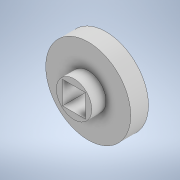
# Autodesk Inventor part: secondwheel
Saved by Autodesk Inventor 2020 (Build 240168000, 168)
## iProperties
Created: 2021-01-09
Part Number: secondwheel
Material: Generic
Document SubType Name: Modeling
Designer: papa
Density: 1 g/cm^3
Appearance: Default
Author: papa
Autodesk Inventor part; units mm, degrees
ref_plane "YZ Plane" through (0, 0, 0) normal (1, 0, 0) x (0, 1, 0)
ref_plane "XZ Plane" through (0, 0, 0) normal (0, 1, 0) x (-1, 0, 0)
ref_plane "XY Plane" through (0, 0, 0) normal (0, 0, 1) x (1, 0, 0)
sketch "Sketch1" plane through (0, 0, 0) normal (0, 0, 1) x (1, 0, 0)
  circle A0 centre (0, 0) radius 12
  line L0 (-3.25, 3.25) -> (3.25, 3.25)
  line L1 (3.25, 3.25) -> (3.25, -3.25)
  line L2 (3.25, -3.25) -> (-3.25, -3.25)
  line L3 (-3.25, -3.25) -> (-3.25, 3.25)
  dimension "d0" = 24
  dimension "d1" = 6.5
  constraints: 8 end point, 2 coincident, 1 centre point, 9 other
  measures "d0" diameter of A0
  measures "d1" distance of L0.start L0.end
extrude "Extrusion1" add sketch "Sketch1" along normal blind 5
sketch "Sketch2" plane through (0, 0, 5) normal (0, 0, 1) x (1, 0, 0)
  circle A0 centre (0, 0) radius 5
  line L0 (-3.25, 3.25) -> (3.25, 3.25) projected
  line L1 (3.25, 3.25) -> (3.25, -3.25)
  line L2 (3.25, -3.25) -> (-3.25, -3.25)
  line L3 (-3.25, -3.25) -> (-3.25, 3.25)
  line L4 (-3.25, 3.25) -> (3.25, 3.25)
  point P0 (0, 3.25)
  constraints: 8 end point, 2 coincident, 2 midpoint, 1 centre point, 9 other
extrude "Extrusion2" add sketch "Sketch2" along normal blind 4
body "Solid1"
